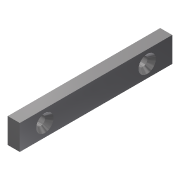
# Autodesk Inventor part: JAW CAP
Saved by Autodesk Inventor 2014 (Build 180170000, 170)
## iProperties
Created: 2014-12-22
Part Number: JAW CAP
Material: Steel, Alloy
Document SubType Name: Modeling
Designer: Ebrahim
Density: 7.85 g/cm^3
Appearance: Semi-Polished
Mass: 340.977 g
Surface Area: 121.795 cm^2
Volume: 43.4365 cm^3
Author: Ebrahim
Autodesk Inventor part; units mm, degrees
ref_plane "YZ Plane" through (0, 0, 0) normal (1, 0, 0) x (0, 1, 0)
ref_plane "XZ Plane" through (0, 0, 0) normal (0, 1, 0) x (-1, 0, 0)
ref_plane "XY Plane" through (0, 0, 0) normal (0, 0, 1) x (1, 0, 0)
sketch "Sketch1" plane through (0, 0, 0) normal (1, 0, 0) x (0, 1, 0)
  line L0 (-76, 12.5) -> (76, 12.5)
  line L1 (76, 12.5) -> (76, -12.5)
  line L2 (76, -12.5) -> (-76, -12.5)
  line L3 (-76, -12.5) -> (-76, 12.5)
  line L4 (-85.317, 0) -> (85.317, 0) construction
  point P0 (0, 0)
  point P1 (0, 0)
  point P2 (-51, 0)
  point P3 (51, 0)
  dimension "d0" = 152
  dimension "d1" = 25
  dimension "d2" = 76
  dimension "d3" = 12.5
  dimension "d4" = 25
  dimension "d5" = 25
  constraints: 10 end point, 2 parallel, 2 perpendicular, 2 point on line, 1 coincident, 1 horizontal, 1 midpoint
  measures "d0" distance of L0.start L0.end
  measures "d1" distance of L0.end L1.end
  measures "d2" distance from line of point (0, 0) L1
  measures "d3" distance from line of point (0, 0) L0
  measures "d4" distance from line of point (-51, 0) L3
  measures "d5" distance from line of point (51, 0) L1
extrude "Extrusion1" add sketch "Sketch1" against normal blind 12
hole "Hole1" at (0, -51, 0) at (0, 51, 0) direction (-1, 0, 0) diameter 9 end through all countersink diameter 17.3 countersink angle 90 clearance for "Countersunk Flat Head Screw ISO 2009/7046" size "M8" standard "ISO"
equation "\"d2\" = 0.5 * d0"
equation "\"d3\" = 0.5 * d1"
body "Solid1"
